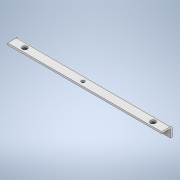
# Autodesk Inventor part: Soporte en L Frontal
Saved by Autodesk Inventor 2020 (Build 240168000, 168)
## iProperties
Created: 2020-06-28
Part Number: Soporte en L Frontal
Material: Aluminum 1100-H14
Document SubType Name: Modelado
Designer: Pipi
Density: 2.7 g/cm^3
Appearance: Satin
Sheet Metal Rule: Por defecto
Author: Pipi
Autodesk Inventor part; units mm, degrees
ref_plane "YZ Plane" through (0, 0, 0) normal (1, 0, 0) x (0, 1, 0)
ref_plane "XZ Plane" through (0, 0, 0) normal (0, 1, 0) x (-1, 0, 0)
ref_plane "XY Plane" through (0, 0, 0) normal (0, 0, 1) x (1, 0, 0)
sketch "Boceto5" plane through (0, 0, 0) normal (0, 1, 0) x (-1, 0, 0)
  line L0 (10.2966, 28.3637) -> (10.2966, 8.3637)
  line L1 (10.2966, 8.3637) -> (-169.7034, 8.3637)
  line L2 (-169.7034, 8.3637) -> (-169.7034, 28.3637)
  line L3 (-169.7034, 28.3637) -> (10.2966, 28.3637)
  line L4 (10.2966, 18.3637) -> (-169.7034, 18.3637)
  circle A0 centre (-154.7034, 23.3637) radius 3
  circle A1 centre (-4.7034, 23.3637) radius 3
  circle A2 centre (-14.7034, 13.3637) radius 3
  circle A3 centre (-144.7034, 13.3637) radius 3
  circle A4 centre (-72.7034, 23.3637) radius 2
  point P0 (0, 0)
  dimension "d33" = 20
  dimension "d34" = 180
  dimension "d35" = 20
  dimension "d36" = 6
  dimension "d37" = 6
  dimension "d38" = 6
  dimension "d39" = 6
  dimension "d40" = 150
  dimension "d41" = 130
  dimension "d42" = 15
  dimension "d43" = 25
  dimension "d44" = 5
  dimension "d45" = 5
  dimension "d46" = 5
  dimension "d47" = 5
  dimension "d54" = 4
  dimension "d56" = 5
  dimension "d57" = 83
  constraints: 10 end point, 5 centre point, 2 midpoint, 2 perpendicular, 1 vertical
  measures "d33" distance of L0.start L0.end
  measures "d34" distance of L0.end L1.end
  measures "d35" distance of L1.end L2.end
  measures "d36" diameter of A0
  measures "d37" diameter of A1
  measures "d38" diameter of A2
  measures "d39" diameter of A3
  measures "d40" distance of A1.centre A0.centre
  measures "d41" distance of A3.centre A2.centre
  measures "d42" distance from line of L0 A1.centre
  measures "d43" distance from line of L0 A2.centre
  measures "d44" distance from line of L1 A3.centre
  measures "d45" distance from line of L1 A2.centre
  measures "d46" distance from line of L3 A1.centre
  measures "d47" distance from line of L3 A0.centre
  measures "d54" diameter of A4
  measures "d56" distance from line of L3 A4.centre
  measures "d57" horizontal distance of L0.start A4.centre
extrude "Extrusión4" add sketch "Boceto5" along normal blind 2 contours L0 L1 L2 L4
extrude "Extrusión5" add sketch "Boceto5" along normal blind 2 contours L0 L4 L2 L3
bend part "Pieza de plegado1" radius 0.5 angle 90 line through (-10.2966, 0, 18.3637) along (1, 0, 0) centre toward (0, -1, 0) moving side (0, 0, -1) both sides no
equation "\"Radio_pliegue\" = Grosor"
equation "\"Anchura_desahogo_plegado\" = Grosor"
equation "\"Profundidad_desahogo_plegado\" = 0.5 * Grosor"
equation "\"Tamaño_destalonado\" = 4 * Grosor"
equation "\"Remanente_mínimo\" = 2 * Grosor"
equation "\"Radiodetransición\" = Radio_pliegue"
equation "\"Tamaño_de_radio_de_Jacobi\" = Grosor"
equation "\"TamañoSeparación\" = Grosor"
equation "\"Grosor\" = 0.5"
